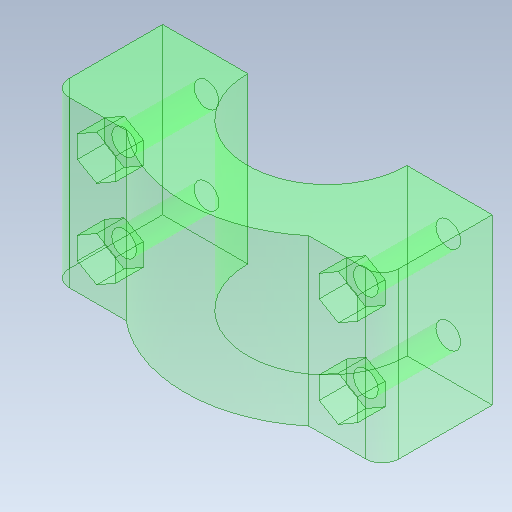
# Autodesk Inventor part: 3_Connettore_inf_INF
Saved by Autodesk Inventor 2020 (Build 240168000, 168)
## iProperties
Created: 2019-10-11
Part Number: 3_Connettore_inf_INF
Material: Generico
Document SubType Name: Modeling
Designer: socci
Density: 1 g/cm^3
Appearance: Verde
Author: socci
Autodesk Inventor part; units mm, degrees
ref_plane "YZ Plane" through (0, 0, 0) normal (1, 0, 0) x (0, 1, 0)
ref_plane "XZ Plane" through (0, 0, 0) normal (0, 1, 0) x (-1, 0, 0)
ref_plane "XY Plane" through (0, 0, 0) normal (0, 0, 1) x (1, 0, 0)
sketch "Schizzo1" plane through (0, 0, 0) normal (0, 0, 1) x (1, 0, 0)
  line L0 (-30, -15) -> (30, -15)
  line L1 (30, -15) -> (30, 15)
  line L2 (30, 15) -> (-30, 15)
  line L3 (-30, 15) -> (-30, -15)
  line L4 (-30, -15) -> (30, 15) construction
  line L5 (30, -15) -> (-30, 15) construction
  point P0 (0, 0)
  point P1 (0, 0)
  dimension "d27" = 30
  dimension "d28" = 60
  constraints: 12 end point, 3 midpoint, 2 parallel, 1 horizontal, 1 perpendicular
  measures "d27" distance of L0.end L1.end
  measures "d28" distance of L0.start L0.end
extrude "Estrusione1" add sketch "Schizzo1" against normal blind 20
sketch "Schizzo2" plane through (-25, 15, 0) normal (0, 1, 0) x (1, 0, 0)
  line L0 (55, 20) -> (-5, 20) projected
  circle A0 centre (25, 20) radius 14.5
  point P0 (25, 0)
  dimension "d60" = 29
  dimension "d61" = 20
  constraints: 1 centre point, 1 coincident, 1 midpoint
  measures "d60" diameter of A0
  measures "d61" distance of point (25, 0) A0.centre
extrude "Estrusione2" cut sketch "Schizzo2" against normal blind 30
sketch "Schizzo6" plane through (0, 0, 0) normal (0, 0, 1) x (1, 0, 0)
  line L0 (0, 15) -> (0, 8)
  line L1 (0, 8) -> (-22, 8)
  line L2 (-22, 8) -> (-22, -8)
  line L3 (0, 8) -> (22, 8)
  line L4 (0, 8) -> (22, 8) construction
  line L5 (22, 8) -> (22, -8)
  point P0 (0, 0)
  dimension "d29" = 7
  dimension "d30" = 22
  dimension "d31" = 90
  dimension "d32" = 16
  dimension "d33" = 90
  dimension "d34" = 22
  dimension "d36" = 16
  dimension "d37" = 90
  constraints: 12 end point, 3 perpendicular, 2 horizontal, 1 collinear, 1 vertical
  measures "d29" distance of L0.start L0.end
  measures "d30" distance of L0.end L1.end
  measures "d31" angle of L0 L1
  measures "d32" distance of L1.end L2.end
  measures "d33" angle of L2 L1
  measures "d34" distance of L0.end L3.end
  measures "d36" distance of L3.end L5.end
  measures "d37" angle of L3 L5
hole "Foro3" at (-22, 8, 0) at (-22, -8, 0) at (22, -8, 0) at (22, 8, 0) direction (0, 0, -1) diameter 4.5 end through all clearance for "Vite a testa piana" size "M4" standard "ANSI - Profilo M Metrico"
sketch "Schizzo7" plane through (0, 0, 0) normal (0, 0, 1) x (1, 0, 0)
  line L0 (-14.5, 15) -> (14.5, 15)
  line L1 (0, 15) -> (0, 8)
  line L2 (0, 8) -> (-22, 8)
  line L3 (-22, 8) -> (-22, -8)
  line L4 (0, 8) -> (22, 8)
  line L5 (0, 8) -> (22, 8) construction
  line L6 (22, 8) -> (22, -8)
  circle A0 centre (-22, 8) radius 3.5
  circle A1 centre (-22, -8) radius 3.5
  circle A2 centre (22, 8) radius 3.5
  circle A3 centre (22, -8) radius 3.5
  line L7 (-18.5, 5.9793) -> (-22, 3.9585)
  line L8 (-22, 3.9585) -> (-25.5, 5.9793)
  line L9 (-25.5, 5.9793) -> (-25.5, 10.0207)
  line L10 (-25.5, 10.0207) -> (-22, 12.0415)
  line L11 (-22, 12.0415) -> (-18.5, 10.0207)
  line L12 (-18.5, 10.0207) -> (-18.5, 5.9793)
  line L13 (-18.5, -10.0207) -> (-22, -12.0415)
  line L14 (-22, -12.0415) -> (-25.5, -10.0207)
  line L15 (-25.5, -10.0207) -> (-25.5, -5.9793)
  line L16 (-25.5, -5.9793) -> (-22, -3.9585)
  line L17 (-22, -3.9585) -> (-18.5, -5.9793)
  line L18 (-18.5, -5.9793) -> (-18.5, -10.0207)
  line L19 (18.5, 10.0207) -> (22, 12.0415)
  line L20 (22, 12.0415) -> (25.5, 10.0207)
  line L21 (25.5, 10.0207) -> (25.5, 5.9793)
  line L22 (25.5, 5.9793) -> (22, 3.9585)
  line L23 (22, 3.9585) -> (18.5, 5.9793)
  line L24 (18.5, 5.9793) -> (18.5, 10.0207)
  line L25 (18.5, -5.9793) -> (22, -3.9585)
  line L26 (22, -3.9585) -> (25.5, -5.9793)
  line L27 (25.5, -5.9793) -> (25.5, -10.0207)
  line L28 (25.5, -10.0207) -> (22, -12.0415)
  line L29 (22, -12.0415) -> (18.5, -10.0207)
  line L30 (18.5, -10.0207) -> (18.5, -5.9793)
  circle A4 centre (-22, 8) radius 2.25 projected
  point P0 (0, 0)
  point P1 (0, 0)
  point P2 (-18.5, 8)
  point P3 (-18.5, -8)
  point P4 (18.5, 8)
  point P5 (18.5, -8)
  dimension "d53" = 7
  dimension "d54" = 7
  dimension "d55" = 7
  dimension "d56" = 7
  dimension "d45" = 7
  dimension "d46" = 22
  dimension "d47" = 90
  dimension "d48" = 16
  dimension "d49" = 90
  dimension "d50" = 22
  dimension "d51" = 16
  dimension "d52" = 90
  constraints: 62 end point, 8 coincident, 5 midpoint, 4 horizontal alignment, 4 point on line, 3 perpendicular, 2 horizontal, 1 collinear, 1 vertical, 61 other
  measures "d45" distance of L1.start L1.end
  measures "d46" distance of L1.end L2.end
  measures "d47" angle of L1 L2
  measures "d48" distance of L2.end L3.end
  measures "d49" angle of L3 L2
  measures "d50" distance of L1.end L4.end
  measures "d51" distance of L4.end L6.end
  measures "d52" angle of L4 L6
extrude "Estrusione4" cut sketch "Schizzo7" against normal blind 5
fillet "Raccordo1" radius 3 1 edges at (30, 0, 0)
fillet "Raccordo2" radius 3 1 edges at (-30, 0, 0)
sketch "Schizzo9" plane through (0, 15, -20) normal (0, 1, 0) x (1, 0, 0)
  circle A0 centre (0, 0) radius 26
  line L0 (27, -20) -> (-27, -20) projected
  line L1 (16.6132, -20) -> (-16.6132, -20)
  point P0 (0, -20)
  dimension "d66" = 52
  constraints: 2 end point, 2 point on circle, 2 point on line, 1 centre point
  measures "d66" diameter of A0
extrude "Estrusione5" add sketch "Schizzo9" against normal blind 30 contours L0 A0 picked at (-3.8639, -21.091)
